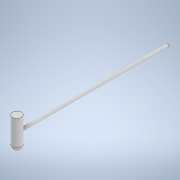
# Autodesk Inventor part: Threaded hammer
Saved by Autodesk Inventor 2021 (Build 250183000, 183)
## iProperties
Created: 2021-02-17
Part Number: Threaded hammer
Material: Generic
Document SubType Name: Modeling
Designer: negt20
Density: 1 g/cm^3
Appearance: Default
Author: negt20
Autodesk Inventor part; units mm, degrees
ref_plane "YZ Plane" through (0, 0, 0) normal (1, 0, 0) x (0, 1, 0)
ref_plane "XZ Plane" through (0, 0, 0) normal (0, 1, 0) x (-1, 0, 0)
ref_plane "XY Plane" through (0, 0, 0) normal (0, 0, 1) x (1, 0, 0)
sketch "Sketch1" plane through (0, 0, 0) normal (0, 0, 1) x (1, 0, 0)
  circle A0 centre (0, 0) radius 2.5
  dimension "d0" = 5
  constraints: 1 centre point, 1 coincident
  measures "d0" diameter of A0
extrude "Extrusion1" add sketch "Sketch1" along normal blind 250
sketch "Sketch2" plane through (0, 0, 250) normal (0, 0, 1) x (1, 0, 0)
  circle A0 centre (0, 0) radius 2.5 projected
  line L0 (0, 0) -> (0, -25)
  line L1 (0, 0) -> (0, 25)
  line L2 (0, 25) -> (7.5, 25)
  line L3 (7.5, 25) -> (7.5, -25)
  line L4 (7.5, -25) -> (0, -25)
  point P0 (0, 0)
  dimension "d12" = 25
  dimension "d14" = 25
  dimension "d15" = 7.5
  constraints: 10 end point, 1 coincident, 1 horizontal, 1 perpendicular, 1 vertical
  measures "d12" distance of L0.start L0.end
  measures "d14" distance of L0.start L1.end
  measures "d15" distance of L1.end L2.end
revolve "Revolution1" add sketch "Sketch2" angle 360 about axis through (0, 0, 250) along (0, 1, 0) picked at (1.6458, -0.1854) contours A0 L0 L1 | A0 L1 L2 L3 L4 L0
fillet "Fillet4" radius 7.5 1 edges at (-7.5, -25, 250)
body "Solid1"
